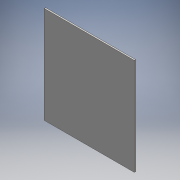
# Autodesk Inventor part: Side_board
Saved by Autodesk Inventor 2016 (Build 200138000, 138)
## iProperties
Created: 2016-11-14
Part Number: Side_board
Material: 一般
Document SubType Name: Modeling
Designer: 宏太
Density: 1 g/cm^3
Appearance: 既定
Author: 宏太
Autodesk Inventor part; units mm, degrees
ref_plane "YZ Plane" through (0, 0, 0) normal (1, 0, 0) x (0, 1, 0)
ref_plane "XZ Plane" through (0, 0, 0) normal (0, 1, 0) x (-1, 0, 0)
ref_plane "XY Plane" through (0, 0, 0) normal (0, 0, 1) x (1, 0, 0)
sketch "スケッチ1" plane through (0, 0, 0) normal (0, 1, 0) x (-1, 0, 0)
  line L0 (0, 0) -> (130, 0)
  line L1 (130, 0) -> (130, 140)
  line L2 (130, 140) -> (0, 140)
  line L3 (0, 140) -> (0, 0)
  dimension "d0" = 130
  dimension "d1" = 140
  constraints: 8 end point, 2 parallel, 1 horizontal, 1 perpendicular
  measures "d0" distance of L2.end L1.end
  measures "d1" distance of L0.end L1.end
extrude "押し出し1" add sketch "スケッチ1" along normal blind 2
